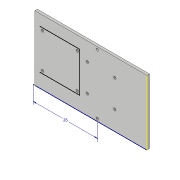
# Autodesk Inventor part: BASE FOR SYSTEM
Saved by Autodesk Inventor 2019 (Build 230136000, 136)
## iProperties
Created: 2019-10-13
Part Number: BASE FOR SYSTEM
Material: Generic
Document SubType Name: Modeling
Designer: Admin
Density: 1 g/cm^3
Appearance: Default
Author: Admin
Autodesk Inventor part; units mm, degrees
ref_plane "YZ Plane" through (0, 0, 0) normal (1, 0, 0) x (0, 1, 0)
ref_plane "XZ Plane" through (0, 0, 0) normal (0, 1, 0) x (-1, 0, 0)
ref_plane "XY Plane" through (0, 0, 0) normal (0, 0, 1) x (1, 0, 0)
sketch "Sketch1" plane through (0, 0, 0) normal (0, 0, 1) x (1, 0, 0)
  line L0 (0, 0) -> (350, 0)
  line L1 (350, 0) -> (350, 260)
  line L2 (350, 260) -> (0, 260)
  line L3 (0, 260) -> (0, 0)
  line L4 (212.725, 66.675) -> (332.725, 66.675)
  line L5 (332.725, 66.675) -> (332.725, 186.675)
  line L6 (332.725, 186.675) -> (212.725, 186.675)
  line L7 (212.725, 186.675) -> (212.725, 66.675)
  circle A0 centre (212.725, 66.675) radius 5
  circle A1 centre (212.725, 186.675) radius 5
  circle A2 centre (332.725, 186.675) radius 5
  circle A3 centre (332.725, 66.675) radius 5
  dimension "d0" = 350
  dimension "d1" = 260
  dimension "d59" = 120
  dimension "d60" = 120
  dimension "d61" = 10
  dimension "d62" = 10
  dimension "d63" = 10
  dimension "d64" = 10
  constraints: 16 end point, 4 centre point, 4 coincident, 4 parallel, 2 horizontal, 2 perpendicular
  measures "d0" distance of L2.end L1.end
  measures "d1" distance of L1.end L0.end
  measures "d59" distance of L6.end L5.end
  measures "d60" distance of L5.end L4.end
  measures "d61" diameter of A0
  measures "d62" diameter of A1
  measures "d63" diameter of A2
  measures "d64" diameter of A3
extrude "Extrusion1" add sketch "Sketch1" along normal blind 10 contours L3 L2 L1 L0 | L7 A0 L4 | L4 A0 L7 | A0 L7 A1 L6 A2 L5 A3 L4 | A3 L5 L4 | L4 L5 A3 | A1 L6 L7 | L7 L6 A1 | A2 L6 L5 | L5 L6 A2
sketch "Sketch2" plane through (0, 0, 10) normal (0, 0, 1) x (1, 0, 0)
  line L0 (0, 0) -> (0, 45)
  line L1 (0, 260) -> (0, 0) projected
  line L2 (0, 260) -> (0, 215)
  line L3 (0, 215) -> (20, 215)
  line L4 (0, 45) -> (20, 45)
  line L5 (20, 45) -> (20, 215)
  dimension "d4" = 45
  dimension "d5" = 45
  dimension "d6" = 20
  dimension "d7" = 20
  constraints: 10 end point, 2 point on line, 1 horizontal, 1 perpendicular
  measures "d4" distance of L0.start L0.end
  measures "d5" distance of L1.start L2.end
  measures "d6" distance of L2.end L3.end
  measures "d7" distance of L0.end L4.end
sketch "Sketch3" plane through (0, 0, 10) normal (0, 0, 1) x (1, 0, 0)
  point P0 (0, 0)
sketch "Sketch4" plane through (0, 0, 10) normal (0, 0, 1) x (1, 0, 0)
  line L0 (0, 0) -> (180, 0)
  line L1 (0, 0) -> (350, 0) projected
  dimension "d8" = 180
  constraints: 2 end point, 1 point on line
  measures "d8" distance of L0.start L0.end
sketch "Sketch5" plane through (0, 0, 10) normal (0, 0, 1) x (1, 0, 0)
  line L0 (19.05, 215.9) -> (179.05, 215.9)
  line L1 (179.05, 215.9) -> (179.05, 55.9)
  line L2 (179.05, 55.9) -> (19.05, 55.9)
  line L3 (19.05, 215.9) -> (38.1, 215.9)
  point P0 (0, 0)
  dimension "d9" = 160
  dimension "d10" = 160
  dimension "d11" = 160
  constraints: 8 end point, 2 perpendicular, 1 horizontal, 1 point on line
  measures "d9" distance of L0.start L0.end
  measures "d10" distance of L0.end L1.end
  measures "d11" distance of L1.end L2.end
sketch "Sketch6" plane through (0, 0, 10) normal (0, 0, 1) x (1, 0, 0)
  line L0 (20.6375, 215.9) -> (30.6375, 215.9)
  line L1 (30.6375, 215.9) -> (30.6375, 65.9)
  line L2 (30.6375, 65.9) -> (170.6375, 65.9)
  line L3 (170.6375, 65.9) -> (170.6375, 205.9)
  line L4 (170.6375, 205.9) -> (30.6375, 205.9)
  circle A0 centre (30.6375, 205.9) radius 5
  circle A1 centre (170.6375, 205.9) radius 5
  circle A2 centre (30.6375, 65.9) radius 5
  circle A3 centre (170.6375, 65.9) radius 5
  line L5 (212.725, 74.6125) -> (332.725, 74.6125)
  line L6 (332.725, 74.6125) -> (332.725, 194.6125)
  line L7 (332.725, 194.6125) -> (212.725, 194.6125)
  line L8 (212.725, 194.6125) -> (212.725, 74.6125)
  circle A4 centre (212.725, 74.6125) radius 5
  circle A5 centre (212.725, 194.6125) radius 5
  circle A6 centre (332.725, 194.6125) radius 5
  circle A7 centre (332.725, 74.6125) radius 5
  point P0 (0, 0)
  dimension "d12" = 10
  dimension "d13" = 150
  dimension "d14" = 140
  dimension "d15" = 140
  dimension "d16" = 140
  dimension "d17" = 10
  dimension "d18" = 10
  dimension "d19" = 10
  dimension "d20" = 10
  dimension "d65" = 120
  dimension "d66" = 120
  dimension "d67" = 10
  dimension "d68" = 10
  dimension "d69" = 10
  dimension "d70" = 10
  constraints: 18 end point, 8 centre point, 8 coincident, 4 perpendicular, 2 horizontal, 2 parallel, 1 point on line
  measures "d12" distance of L0.start L0.end
  measures "d13" distance of L0.end L1.end
  measures "d14" distance of L1.end L2.end
  measures "d15" distance of L2.end L3.end
  measures "d16" distance of L3.end L4.end
  measures "d17" diameter of A0
  measures "d18" diameter of A1
  measures "d19" diameter of A2
  measures "d20" diameter of A3
  measures "d65" distance of L7.end L6.end
  measures "d66" distance of L6.end L5.end
  measures "d67" diameter of A4
  measures "d68" diameter of A5
  measures "d69" diameter of A6
  measures "d70" diameter of A7
extrude "Extrusion2" cut sketch "Sketch6" along normal through all both and the other way through all contours A0 L4 L1 | L1 A0 | L4 A0 L1 | A1 L3 L4 | L4 L3 A1 | A2 L2 L1 | L1 L2 A2 | A3 L2 L3 | L3 L2 A3
sketch "Sketch7" plane through (0, 0, 10) normal (0, 0, 1) x (1, 0, 0)
  circle A0 centre (170.6375, 65.9) radius 5 projected
  line L0 (170.6375, 65.9) -> (190.6375, 65.9)
  line L1 (190.6375, 65.9) -> (190.6375, 225.9)
  line L2 (190.6375, 225.9) -> (190.6375, 204.7875)
  point P0 (0, 0)
  dimension "d23" = 20
  dimension "d24" = 160
  constraints: 6 end point, 1 horizontal, 1 perpendicular, 1 point on line
  measures "d23" distance of L0.start L0.end
  measures "d24" distance of L0.end L1.end
sketch "Sketch8" plane through (0, 0, 10) normal (0, 0, 1) x (1, 0, 0)
  line L0 (171.45, 204.7875) -> (190.5, 204.7875)
  line L1 (190.5, 204.7875) -> (190.5, 179.7875)
  point P0 (0, 0)
  dimension "d45" = 25
  constraints: 4 end point, 1 vertical
  measures "d45" distance of L0.end L1.end
extrude "Extrusion3" [suppressed]
sketch "Sketch9" plane through (0, 0, 10) normal (0, 0, 1) x (1, 0, 0)
  point P0 (0, 0)
sketch "Sketch10" plane through (0, 0, 0) normal (0, 0, -1) x (-1, 0, 0)
  line L0 (-211.1375, 187.325) -> (-321.1375, 187.325)
  line L1 (-321.1375, 187.325) -> (-321.1375, 77.325)
  line L2 (-321.1375, 77.325) -> (-211.1375, 77.325)
  line L3 (-211.1375, 77.325) -> (-211.1375, 187.325)
  circle A0 centre (-211.1375, 187.325) radius 5
  circle A1 centre (-211.1375, 77.325) radius 5
  circle A2 centre (-321.1375, 77.325) radius 5
  circle A3 centre (-321.1375, 187.325) radius 5
  point P0 (0, 0)
  dimension "d71" = 110
  dimension "d72" = 110
  dimension "d73" = 10
  dimension "d74" = 10
  dimension "d75" = 10
  dimension "d76" = 10
  constraints: 8 end point, 4 centre point, 4 coincident, 2 parallel, 1 horizontal, 1 perpendicular
  measures "d71" distance of L2.end L1.end
  measures "d72" distance of L1.end L0.end
  measures "d73" diameter of A0
  measures "d74" diameter of A1
  measures "d75" diameter of A2
  measures "d76" diameter of A3
extrude "Extrusion4" cut sketch "Sketch10" against normal through all contours A3 L1 L0 | L0 L1 A3 | A0 L3 L0 | L0 L3 A0 | A2 L2 L1 | L1 L2 A2 | A1 L2 L3 | L3 L2 A1
sketch "Sketch11" plane through (0, 0, 10) normal (0, 0, 1) x (1, 0, 0)
  line L0 (350, 260) -> (450, 260)
  line L1 (450, 260) -> (450, 0)
  line L2 (450, 0) -> (350, 0)
  line L3 (350, 0) -> (350, 260)
  point P0 (0, 0)
  dimension "d79" = 100
  constraints: 8 end point, 2 parallel, 1 horizontal, 1 perpendicular
  measures "d79" distance of L1.end L2.end
extrude "Extrusion5" add sketch "Sketch11" against normal blind 10
sketch "Sketch12" plane through (0, 0, 10) normal (0, 0, 1) x (1, 0, 0)
  point P0 (0, 0)
sketch "Sketch13" plane through (0, 0, 10) normal (0, 0, 1) x (1, 0, 0)
  line L0 (450, 260) -> (450, 0) projected
  line L1 (450, 0) -> (250.825, 0)
  line L2 (0, 0) -> (450, 0) projected
  constraints: 2 end point, 1 point on line
sketch "Sketch14" plane through (0, 0, 10) normal (0, 0, 1) x (1, 0, 0)
  line L0 (0, 0) -> (450, 0) projected
  line L1 (252.4125, 0) -> (252.4125, 20)
  line L2 (450, 0) -> (252.4125, 0)
  line L3 (252.4125, 0) -> (252.4125, 10)
  circle A0 centre (252.4125, 10) radius 5
  line L4 (252.4125, 10) -> (252.4125, 258.7625)
  line L5 (252.4125, 258.7625) -> (252.4125, 248.7625)
  circle A1 centre (252.4125, 248.7625) radius 5
  dimension "d89" = 10
  dimension "d90" = 10
  dimension "d91" = 10
  dimension "d92" = 10
  constraints: 10 end point, 3 point on line, 2 centre point, 2 coincident, 2 perpendicular, 1 midpoint
  measures "d89" distance of L1.start L3.end
  measures "d90" diameter of A0
  measures "d91" distance of L4.end L5.end
  measures "d92" diameter of A1
extrude "Extrusion6" [suppressed]
sketch "Sketch15" plane through (0, 0, 10) normal (0, 0, 1) x (1, 0, 0)
  line L0 (0, 0) -> (450, 0) projected
  line L1 (252.4125, 232.581) -> (252.4125, 242.8875)
  constraints: 2 end point
extrude "Extrusion7" [suppressed]
sketch "Sketch16" plane through (0, 0, 10) normal (0, 0, 1) x (1, 0, 0)
  line L0 (0, 0) -> (450, 0) projected
  line L1 (252.4125, 0) -> (-7.5875, 0)
  dimension "d93" = 260
  constraints: 2 end point, 1 collinear, 1 point on line
  measures "d93" distance of L1.start L1.end
sketch "Sketch17" plane through (0, 0, 10) normal (0, 0, 1) x (1, 0, 0)
  line L0 (250.825, 0) -> (250.825, 10)
  line L1 (250.825, 10) -> (250.825, 250)
  circle A0 centre (250.825, 250) radius 5
  circle A1 centre (250.825, 10) radius 5
  point P0 (0, 0)
  dimension "d94" = 10
  dimension "d95" = 240
  dimension "d96" = 10
  dimension "d97" = 10
  constraints: 4 end point, 2 centre point, 2 coincident, 1 point on line, 1 vertical
  measures "d94" distance of L0.start L0.end
  measures "d95" distance of L0.end L1.end
  measures "d96" diameter of A0
  measures "d97" diameter of A1
extrude "Extrusion8" cut sketch "Sketch17" against normal blind 10
equation "\"d36\" = d29"
equation "\"d98\" = d97"
equation "\"d29\" = 10"
body "Solid1"
